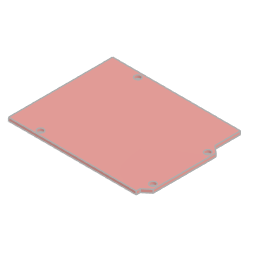
Arduino_UNO_PCB (Autodesk Fusion 360 design; units mm, degrees)
Autodesk Fusion 360 part; units mm, degrees
sketch "Sketch1" plane through (0, 0, 0) normal (0, 0, 1) x (1, 0, 0)
  line L0 (0, 0) -> (65, 0)
  line L1 (65, 0) -> (65, 53)
  line L2 (65, 53) -> (0, 53)
  line L3 (0, 53) -> (0, 0)
  line L4 (65, 2) -> (68.6, 5)
  line L5 (68.6, 5) -> (68.6, 37)
  line L6 (68.6, 37) -> (65, 40)
  circle A0 centre (14, 2.3) radius 1.6
  circle A1 centre (15.3, 50.5) radius 1.6
  circle A2 centre (66.1, 35.3) radius 1.6
  circle A3 centre (66.1, 7.4) radius 1.6
  dimension "d1" = 65
  dimension "d2" = 53
  dimension "d3" = 68.6
  dimension "d4" = 37
  dimension "d5" = 40
  dimension "d6" = 2
  dimension "d7" = 5
  dimension "d8" = 3.2
  dimension "d9" = 15.3
  dimension "d10" = 50.5
  dimension "d11" = 7.4
  dimension "d12" = 35.3
  dimension "d13" = 66.1
  dimension "d14" = 2.3
  dimension "d17" = 14
  constraint horizontal L0
  constraint vertical L1
  constraint horizontal L2
  constraint vertical L3
  constraint coincident L0.start L3.end
  constraint coincident L1 L4.start
  constraint vertical L5
  constraint coincident L1 L6.end
  constraint equal A0 A1
  constraint equal A0 A3
  constraint equal A0 A2
  constraint vertical A2.centre A3.centre
  measures "d1" distance of L0.start L0.end
  measures "d2" distance of L0.start L2.end
  measures "d3" distance of L3 L5
  measures "d4" distance of L0 L5.end
  measures "d5" distance of L0 L6.end
  measures "d6" distance of L0 L4.start
  measures "d7" distance of L0 L4.end
  measures "d8" diameter of A0
  measures "d9" distance of L3 A1.centre
  measures "d10" distance of L0 A1.centre
  measures "d11" distance of L0 A3.centre
  measures "d12" distance of L0 A2.centre
  measures "d13" distance of L3 A3.centre
  measures "d14" distance of L0 A0.centre
  measures "d17" distance of L3 A0.centre
extrude "Extrude1" add sketch "Sketch1" along normal blind 1.7 contours L0 L1 L2 L3 A2 A3 | L1 L4 L5 L6 A2 A3
named bodies: "PCB"
